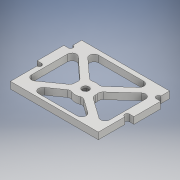
# Autodesk Inventor part: 付け根_サブフレーム_2_3
Saved by Autodesk Inventor 2018 (Build 220112000, 112)
## iProperties
Created: 2018-08-31
Part Number: 付け根_サブフレーム_2_3
Material: アルミニウム 2014-T4
Document SubType Name: Modeling
Designer: taka
Density: 2.8 g/cm^3
Appearance: サテン
Mass: 5.08742 g
Surface Area: 24.069 cm^2
Volume: 1.81694 cm^3
Author: taka
Autodesk Inventor part; units mm, degrees
ref_plane "YZ Plane" through (0, 0, 0) normal (1, 0, 0) x (0, 1, 0)
ref_plane "XZ Plane" through (0, 0, 0) normal (0, 1, 0) x (-1, 0, 0)
ref_plane "XY Plane" through (0, 0, 0) normal (0, 0, 1) x (1, 0, 0)
sketch "スケッチ1" plane through (0, 0, 0) normal (0, 0, 1) x (1, 0, 0)
  circle A0 centre (0, 0) radius 1.55
  circle A1 centre (0, 0) radius 3.1754 construction
  arc A2 (4.2833, 1.8743) -> (2.2625, 4.0915) centre (0, 0) ccw construction
  line L0 (-3.1754, 0) -> (-1.5877, 2.75) construction
  line L1 (-1.5877, 2.75) -> (1.5877, 2.75) construction
  line L2 (1.5877, 2.75) -> (3.1754, 0) construction
  line L3 (3.1754, 0) -> (1.5877, -2.75) construction
  line L4 (1.5877, -2.75) -> (-1.5877, -2.75) construction
  line L5 (-1.5877, -2.75) -> (-3.1754, 0) construction
  line L6 (-19.75, 18) -> (19.75, 18)
  line L7 (19.75, 18) -> (19.75, 14.1)
  line L8 (19.75, -14) -> (-19.75, -14)
  line L9 (0, 0) -> (0, -14) construction
  line L10 (19.75, 12) -> (21.75, 12)
  line L11 (21.75, 12) -> (21.75, 0)
  line L12 (21.75, 0) -> (19.75, 0)
  line L13 (19.75, 0) -> (19.75, 12) construction
  arc A3 (19.75, 14.1) -> (19.75, 12) centre (19.75, 13.05) ccw
  arc A4 (19.75, 0) -> (19.75, -2.1) centre (19.75, -1.05) ccw
  line L14 (19.75, 14.1) -> (19.75, 12) construction
  line L15 (19.75, 12) -> (19.75, 0) construction
  line L16 (19.75, 0) -> (19.75, -2.1) construction
  line L17 (19.75, -2.1) -> (19.75, -14)
  line L18 (-19.75, 18) -> (-19.75, 14.1)
  line L19 (-19.75, 12) -> (-21.75, 12)
  line L20 (-21.75, 12) -> (-21.75, 0)
  line L21 (-21.75, 0) -> (-19.75, 0)
  line L22 (-19.75, 0) -> (-19.75, 12) construction
  arc A5 (-19.75, 12) -> (-19.75, 14.1) centre (-19.75, 13.05) ccw
  arc A6 (-19.75, -2.1) -> (-19.75, 0) centre (-19.75, -1.05) ccw
  line L23 (-19.75, 14.1) -> (-19.75, 12) construction
  line L24 (-19.75, 12) -> (-19.75, 0) construction
  line L25 (-19.75, 0) -> (-19.75, -2.1) construction
  line L26 (-19.75, -2.1) -> (-19.75, -14)
  line L27 (-19.75, 18) -> (0, 0) construction
  line L28 (0, 0) -> (19.75, -14) construction
  line L29 (0, 0) -> (-19.75, -14) construction
  line L30 (0, 0) -> (19.75, 18) construction
  line L31 (-17.5556, 16) -> (-15.3287, 16) construction
  line L32 (17.5556, 16) -> (17.5556, 13.9705) construction
  line L33 (17.5556, -12.4444) -> (14.9618, -12.4444) construction
  line L34 (-17.5556, -12.4444) -> (-17.5556, -10.6058) construction
  line L35 (-15.3287, 16) -> (-2.2625, 4.0915)
  line L36 (-4.2833, 1.8743) -> (-17.5556, 13.9705)
  line L37 (-4.4801, -1.3372) -> (-17.5556, -10.6058)
  line L38 (-2.7452, -3.7846) -> (-14.9618, -12.4444)
  line L39 (-15.3287, 16) -> (15.3287, 16)
  line L40 (-17.5556, 13.9705) -> (-17.5556, 16) construction
  line L41 (-17.5556, -10.6058) -> (-17.5556, 13.9705)
  line L42 (-14.9618, -12.4444) -> (-17.5556, -12.4444) construction
  line L43 (15.3287, 16) -> (2.2625, 4.0915)
  line L44 (4.2833, 1.8743) -> (17.5556, 13.9705)
  line L45 (4.4801, -1.3372) -> (17.5556, -10.6058)
  line L46 (2.7452, -3.7846) -> (14.9618, -12.4444)
  line L47 (15.3287, 16) -> (17.5556, 16) construction
  line L48 (17.5556, 13.9705) -> (17.5556, -10.6058)
  line L49 (17.5556, -10.6058) -> (17.5556, -12.4444) construction
  line L50 (14.9618, -12.4444) -> (-14.9618, -12.4444)
  arc A7 (4.4801, -1.3372) -> (4.2833, 1.8743) centre (0, 0) ccw
  arc A8 (2.2625, 4.0915) -> (-2.2625, 4.0915) centre (0, 0) ccw
  arc A9 (-2.2625, 4.0915) -> (-4.2833, 1.8743) centre (0, 0) ccw construction
  arc A10 (-4.2833, 1.8743) -> (-4.4801, -1.3372) centre (0, 0) ccw
  arc A11 (-4.4801, -1.3372) -> (-2.7452, -3.7846) centre (0, 0) ccw construction
  arc A12 (-2.7452, -3.7846) -> (2.7452, -3.7846) centre (0, 0) ccw
  arc A13 (2.7452, -3.7846) -> (4.4801, -1.3372) centre (0, 0) ccw construction
  dimension "d1" = 3.1
  dimension "d3" = 1.5
  dimension "d4" = 5.5
  dimension "d6" = 32
  dimension "d7" = 18
  dimension "d8" = 2
  dimension "d9" = 12
  dimension "d10" = 2.1
  dimension "d11" = 2.1
  dimension "d12" = 39.5
  dimension "d13" = 6
  dimension "d15" = 2
  dimension "d16" = 1.5
  dimension "d17" = 1.5
  dimension "d18" = 1.5
  dimension "d19" = 1.5
  constraints: 102 end point, 34 point on circle, 25 parallel, 19 point on line, 16 perpendicular, 16 symmetric about line, 13 centre point, 5 coincident, 5 horizontal, 5 midpoint, 2 tangent, 1 horizontal alignment, 18 other
  measures "d1" diameter of A0
  measures "d4" distance of L3.end L1.end
  measures "d6" distance between parallel lines of L8 L6
  measures "d7" distance from line of point (0, 0) L6
  measures "d8" distance of L11.end L12.end
  measures "d9" distance of L10.end L11.end
  measures "d10" diameter of A3
  measures "d11" diameter of A4
  measures "d12" distance between parallel lines of L17 L26
  measures "d13" distance between parallel lines of L6 L10
  measures "d15" distance between parallel lines of L6 L31
  measures "d16" distance between parallel lines of L27 L35
  measures "d17" distance between parallel lines of L36 L27
  measures "d18" distance between parallel lines of L29 L37
  measures "d19" distance between parallel lines of L29 L38
extrude "押し出し1" add sketch "スケッチ1" along normal blind 3
sketch "スケッチ2" plane through (0, 0, 0) normal (0, 0, -1) x (-1, 0, 0)
  circle A0 centre (0, 0) radius 1.55 projected
  line L0 (-2.75, 1.5877) -> (0, 3.1754)
  line L1 (0, 3.1754) -> (2.75, 1.5877)
  line L2 (2.75, 1.5877) -> (2.75, -1.5877)
  line L3 (2.75, -1.5877) -> (0, -3.1754)
  line L4 (0, -3.1754) -> (-2.75, -1.5877)
  line L5 (-2.75, -1.5877) -> (-2.75, 1.5877)
  line L6 (2.8, 1.6166) -> (0, 3.2332)
  line L7 (0, 3.2332) -> (-2.8, 1.6166)
  line L8 (-2.8, 1.6166) -> (-2.8, -1.6166)
  line L9 (-2.8, -1.6166) -> (0, -3.2332)
  line L10 (0, -3.2332) -> (2.8, -1.6166)
  line L11 (2.8, -1.6166) -> (2.8, 1.6166)
  circle A1 centre (0, 2.1832) radius 1.05
  circle A2 centre (-1.8907, 1.0916) radius 1.05
  circle A3 centre (-1.8907, -1.0916) radius 1.05
  circle A4 centre (0, -2.1832) radius 1.05
  circle A5 centre (1.8907, -1.0916) radius 1.05
  circle A6 centre (1.8907, 1.0916) radius 1.05
  line L12 (0, 0) -> (0, -1.55) construction
  point P0 (-2.8, 1.6166)
  point P1 (-2.8, -1.6166)
  point P2 (0, -3.2332)
  point P3 (2.8, -1.6166)
  point P4 (2.8, 1.6166)
  dimension "d24" = 2.1
  dimension "d22" = 5.5
  dimension "d23" = 0.05
  dimension "d27" = 360
  constraints: 26 end point, 3 vertical alignment, 1 coincident, 1 vertical, 55 other
  measures "d22" distance between parallel lines of L2 L5
  measures "d23" distance between parallel lines of L1 L6
extrude "押し出し2" cut sketch "スケッチ2" against normal blind 2 contours A0 A6 L2 A5 | A6 A0 | A0 A6 L1 L2 | A5 L2 L3 A0 | A0 A5 | A0 A1 L1 A6 | L2 L1 A6 L6 L11 | A5 L3 A4 A0 | A5 L11 L10 L3 L2 | A1 A0 | A0 A1 L0 L1 | L11 A6 | A4 L3 L4 A0 | A0 A4 | A5 L11 | A0 A2 L0 A1 | L1 L0 A1 L7 L6 | A6 L6 | A4 L4 A3 A0 | A4 L10 L9 L4 L3 | L10 A5 | A2 A0 | A0 A2 L5 L0 | L6 A1 | A3 L4 L5 A0 | A0 A3 | A4 L10 | A0 A3 L5 A2 | L0 L5 A2 L8 L7 | A1 L7 | A3 L9 L8 L5 L4 | L9 A4 | L7 A2 | A3 L9 | A2 L8 | L8 A3
fillet "フィレット1" radius 2 16 edges at (-4.2833, 1.8743, 1.5) (-4.4801, -1.3372, 1.5) (-2.2625, 4.0915, 1.5) (2.2625, 4.0915, 1.5) (17.5556, -10.6058, 1.5) (-14.9618, -12.4444, 1.5) (14.9618, -12.4444, 1.5) (4.4801, -1.3372, 1.5) (4.2833, 1.8743, 1.5) (-2.7452, -3.7846, 1.5) (2.7452, -3.7846, 1.5) (-17.5556, -10.6058, 1.5) (-17.5556, 13.9705, 1.5) (-15.3287, 16, 1.5) (15.3287, 16, 1.5) (17.5556, 13.9705, 1.5)
equation "\"d17\" = d16"
equation "\"d18\" = d16"
equation "\"d19\" = d16"
